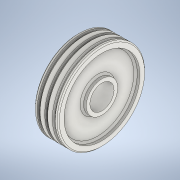
# Autodesk Inventor part: Kolben
Saved by Autodesk Inventor 2020.3 (Build 243373000, 373)
## iProperties
Created: 2021-05-20
Part Number: Kolben
Material: Stahl AISI 4130
Document SubType Name: Modeling
Designer: Preuß P. Ch.
Density: 7.85 g/cm^3
Appearance: Stahl
Author: Preuß P. Ch.
Autodesk Inventor part; units mm, degrees
ref_plane "YZ Plane" through (0, 0, 0) normal (1, 0, 0) x (0, 1, 0)
ref_plane "XZ Plane" through (0, 0, 0) normal (0, 1, 0) x (-1, 0, 0)
ref_plane "XY Plane" through (0, 0, 0) normal (0, 0, 1) x (1, 0, 0)
sketch "Skizze1" plane through (0, 0, 0) normal (0, 0, 1) x (1, 0, 0)
  line L0 (0, 0) -> (41, 0)
  line L1 (41, 0) -> (41, 75)
  line L2 (41, 75) -> (0, 75)
  line L3 (0, 75) -> (0, 0)
  line L4 (5, 75) -> (10, 75)
  line L5 (10, 75) -> (10, 70)
  line L6 (10, 70) -> (5, 70)
  line L7 (5, 70) -> (5, 75)
  line L8 (18, 75) -> (23, 75)
  line L9 (23, 75) -> (23, 70)
  line L10 (23, 70) -> (18, 70)
  line L11 (18, 70) -> (18, 75)
  line L12 (31, 75) -> (36, 75)
  line L13 (36, 75) -> (36, 70)
  line L14 (36, 70) -> (31, 70)
  line L15 (31, 70) -> (31, 75)
  line L16 (0, 65) -> (10, 65)
  line L17 (10, 65) -> (10, 32)
  line L18 (10, 32) -> (0, 32)
  line L19 (0, 32) -> (0, 65)
  line L20 (41, 65) -> (33.5, 65)
  line L21 (33.5, 65) -> (33.5, 27)
  line L22 (33.5, 27) -> (41, 27)
  line L23 (41, 27) -> (41, 65)
  line L24 (41, 20.6907) -> (0, 25)
  point P0 (0, 32)
  dimension "d0" = 150
  dimension "d1" = 41
  dimension "d2" = 5
  dimension "d3" = 5
  dimension "d4" = 5
  dimension "d5" = 18
  dimension "d6" = 31
  dimension "d7" = 64
  dimension "d8" = 54
  dimension "d9" = 130
  dimension "d10" = 130
  dimension "d11" = 7.5
  dimension "d12" = 10
  dimension "d13" = 96
  dimension "d14" = 50
  constraints: 50 end point, 12 parallel, 7 point on line, 6 horizontal, 6 perpendicular, 4 equal length
  measures "d0" diameter of L2 L0
  measures "d1" distance of L0.start L0.end
  measures "d2" distance of L5.end L6.end
  measures "d3" distance of L6.end L4.start
  measures "d4" distance between parallel lines of L7 L3
  measures "d5" distance between parallel lines of L11 L3
  measures "d6" distance between parallel lines of L15 L3
  measures "d7" diameter of L18 L0
  measures "d8" diameter of L22 L0
  measures "d9" diameter of L20 L0
  measures "d10" diameter of L16 L0
  measures "d11" distance of L21.end L22.end
  measures "d12" distance of L17.end L18.end
  measures "d13" angle of L1 L24
  measures "d14" diameter of L24.end L0
revolve "Umdrehung1" add sketch "Skizze1" angle 360 about axis through (0, 0, 0) along (1, 0, 0) contours L3 L18 L17 L16 L2 L7 L6 L5 L11 L10 L9 L15 L14 L13 L1 L20 L21 L22 L24
chamfer "Fase1" distance 3 angle 45 4 edges at (33.5, -65, 0) (33.5, -27, 0) (10, -32, 0) (10, -65, 0)
chamfer "Fase2" distance 2 angle 45 2 edges at (41, -75, 0) (0, -75, 0)
equation "\"d10\" = d9"
